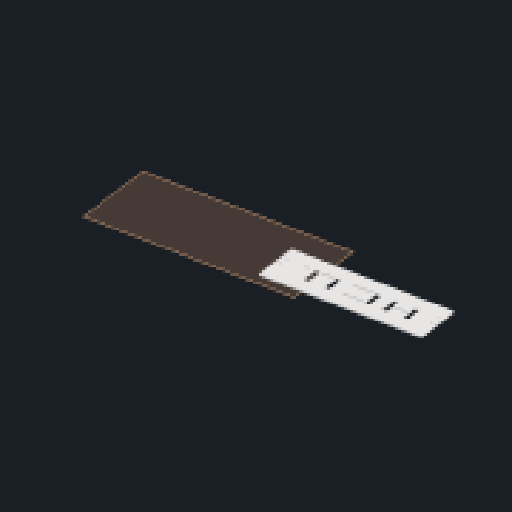
# Autodesk Inventor part: lid
Saved by Autodesk Inventor 2026.1 (Build 301233000, 233)
## iProperties
Created: 2025-08-11
Part Number: lid
Material: Generic
Document SubType Name: Modeling
Designer: jasper
Density: 1 g/cm^3
Appearance: Default
Author: jasper
Autodesk Inventor part; units mm, degrees
ref_plane "YZ Plane" through (0, 0, 0) normal (1, 0, 0) x (0, 1, 0)
ref_plane "XZ Plane" through (0, 0, 0) normal (0, 1, 0) x (-1, 0, 0)
ref_plane "XY Plane" through (0, 0, 0) normal (0, 0, 1) x (1, 0, 0)
ref_plane "Work Plane1" through (-44.2442, 201.0353, -515.4022) normal (0, -0.9118117, 0.4106085) x (-0.1431647, -0.4063788, -0.902419)
sketch "Sketch1" plane through (-44.2442, 201.0353, -515.4022) normal (0, -0.9118117, 0.4106085) x (-0.1431647, -0.4063788, -0.902419)
  circle A0 centre (-31.8295, -172.2882) radius 2.1 projected
  circle A1 centre (-6.35, -6.35) radius 2.1 projected
  circle A2 centre (-31.75, -6.35) radius 2.1 projected
  circle A3 centre (-6.4295, -172.2882) radius 2.1 projected
  circle A4 centre (-31.8295, -172.2882) radius 2.1 projected
  line L0 (50.8, 0) -> (-69.85, 0)
  line L1 (-69.85, 0) -> (-69.85, -178.6382)
  line L2 (-69.85, -178.6382) -> (50.8, -178.6382)
  line L3 (50.8, -178.6382) -> (50.8, 0)
  line L4 (-6.35, -6.35) -> (-31.75, -6.35) construction
  line L5 (-19.05, -6.35) -> (-19.05, -172.2882) construction
  line L6 (-6.4295, -172.2882) -> (-31.8295, -172.2882) construction
  point P0 (-389.7465, -11.674)
  dimension "d41" = 69.85
  dimension "d42" = 50.8
  dimension "d43" = 6.35
  dimension "d44" = 6.35
  constraints: 14 end point, 3 horizontal, 2 parallel, 1 midpoint, 1 perpendicular, 1 point on line, 1 vertical
  measures "d41" distance between parallel lines of L3 L5
  measures "d42" distance between parallel lines of L1 L5
  measures "d43" distance between parallel lines of L4 L0
  measures "d44" distance from line of L2 L6.start
extrude "Extrusion1" add sketch "Sketch1" along normal blind 1.5875
sketch "Sketch2" plane through (-44.2442, 199.5878, -514.7504) normal (0, -0.9118117, 0.4106085) x (-0.9896989, 0.0587846, 0.1305393)
  line L0 (27.0256, 12.7) -> (32.1056, 12.7)
  line L1 (32.1056, 12.7) -> (32.1056, -31.75)
  line L2 (32.1056, -31.75) -> (27.0256, -31.75)
  line L3 (27.0256, -31.75) -> (27.0256, 12.7)
  line L4 (49.8856, 12.7) -> (54.9656, 12.7)
  line L5 (54.9656, 12.7) -> (54.9656, -31.75)
  line L6 (54.9656, -31.75) -> (49.8856, -31.75)
  line L7 (49.8856, -31.75) -> (49.8856, 12.7)
  line L8 (34.6456, -6.985) -> (47.3456, -6.985)
  line L9 (47.3456, -6.985) -> (47.3456, -12.065)
  line L10 (47.3456, -12.065) -> (34.6456, -12.065)
  line L11 (34.6456, -12.065) -> (34.6456, -6.985)
  line L12 (68.9356, 12.7) -> (74.0156, 12.7)
  line L13 (74.0156, 12.7) -> (74.0156, -31.75)
  line L14 (74.0156, -31.75) -> (68.9356, -31.75)
  line L15 (68.9356, -31.75) -> (68.9356, 12.7)
  line L16 (76.5556, 12.7) -> (98.6536, 12.7)
  line L17 (98.6536, 12.7) -> (98.6536, 7.62)
  line L18 (98.6536, 7.62) -> (76.5556, 7.62)
  line L19 (76.5556, 7.62) -> (76.5556, 12.7)
  line L20 (76.5556, -31.75) -> (98.6536, -31.75)
  line L21 (98.6536, -31.75) -> (98.6536, -26.67)
  line L22 (98.6536, -26.67) -> (76.5556, -26.67)
  line L23 (76.5556, -26.67) -> (76.5556, -31.75)
  line L24 (112.6236, 12.7) -> (117.7036, 12.7)
  line L25 (117.7036, 12.7) -> (117.7036, -31.75)
  line L26 (117.7036, -31.75) -> (112.6236, -31.75)
  line L27 (112.6236, -31.75) -> (112.6236, 12.7)
  line L28 (135.4836, 12.7) -> (140.5636, 12.7)
  line L29 (140.5636, 12.7) -> (140.5636, -31.75)
  line L30 (140.5636, -31.75) -> (135.4836, -31.75)
  line L31 (135.4836, -31.75) -> (135.4836, 12.7)
  line L32 (120.2436, -26.67) -> (132.9436, -26.67)
  line L33 (132.9436, -26.67) -> (132.9436, -31.75)
  line L34 (132.9436, -31.75) -> (120.2436, -31.75)
  line L35 (120.2436, -31.75) -> (120.2436, -26.67)
  line L36 (146.5326, -26.67) -> (151.6126, -26.67)
  line L37 (151.6126, -26.67) -> (151.6126, -31.75)
  line L38 (151.6126, -31.75) -> (146.5326, -31.75)
  line L39 (146.5326, -31.75) -> (146.5326, -26.67)
  line L40 (27.0256, -43.4347) -> (151.6126, -43.4347) construction
  line L41 (0, -69.85) -> (178.6382, -69.85) projected
  line L42 (89.3191, -69.85) -> (89.3191, 50.8) construction
  line L43 (178.6382, 50.8) -> (0, 50.8) projected
  line L44 (0, 50.8) -> (0, -69.85) projected
  line L45 (0, -9.525) -> (178.6382, -9.525) construction
  line L46 (178.6382, -69.85) -> (178.6382, 50.8) projected
  point P0 (11.674, -389.7465)
  point P1 (47.3456, -9.525)
  point P2 (34.6456, -9.525)
  point P3 (32.1056, -9.525)
  point P4 (54.9656, -9.525)
  point P5 (132.9436, -29.21)
  point P6 (120.2436, -29.21)
  point P7 (140.5636, -9.525)
  point P8 (89.3191, -43.4347)
  point P9 (12.8847, -9.525)
  dimension "d11" = 5.08
  dimension "d12" = 44.45
  dimension "d13" = 5.08
  dimension "d14" = 44.45
  dimension "d15" = 2.54
  dimension "d16" = 2.54
  dimension "d17" = 12.7
  dimension "d18" = 5.08
  dimension "d19" = 44.45
  dimension "d20" = 13.97
  dimension "d21" = 2.54
  dimension "d22" = 22.098
  dimension "d23" = 5.08
  dimension "d24" = 5.08
  dimension "d25" = 5.08
  dimension "d26" = 44.45
  dimension "d27" = 5.08
  dimension "d28" = 44.45
  dimension "d29" = 2.54
  dimension "d30" = 2.54
  dimension "d31" = 12.7
  dimension "d32" = 5.08
  dimension "d33" = 5.08
  dimension "d34" = 13.97
  dimension "d35" = 5.08
  dimension "d36" = 5.08
  dimension "d37" = 5.969
  constraints: 86 end point, 21 parallel, 12 midpoint, 11 horizontal, 10 perpendicular, 8 collinear, 5 point on line, 2 horizontal alignment
  measures "d11" distance of L0.start L0.end
  measures "d12" distance of L2.end L0.start
  measures "d13" distance of L4.start L4.end
  measures "d14" distance of L6.end L4.start
  measures "d15" distance from line of L7 point (47.346, -9.525)
  measures "d16" distance from line of L1 point (34.646, -9.525)
  measures "d17" distance of L9.end L10.end
  measures "d18" distance of L15.end L13.start
  measures "d19" distance of L14.end L15.end
  measures "d20" distance from line of point (54.966, -9.525) L15
  measures "d21" distance between parallel lines of L13 L19
  measures "d22" distance of L16.start L16.end
  measures "d23" distance of L16.end L17.end
  measures "d24" distance of L20.end L21.end
  measures "d25" distance of L27.end L25.start
  measures "d26" distance of L26.end L27.end
  measures "d27" distance of L28.start L28.end
  measures "d28" distance of L30.end L28.start
  measures "d29" distance from line of L31 point (132.944, -29.21)
  measures "d30" distance from line of L25 point (120.244, -29.21)
  measures "d31" distance of L34.start L34.end
  measures "d32" distance between parallel lines of L34 L32
  measures "d33" distance of L10.end L8.start
  measures "d34" distance between parallel lines of L17 L27
  measures "d35" distance of L36.end L37.end
  measures "d36" distance of L36.start L36.end
  measures "d37" distance between parallel lines of L29 L39
extrude "Extrusion2" cut sketch "Sketch2" against normal blind 1.5875 contours L0 L1 L2 L3 | L4 L5 L6 L7 | L8 L9 L10 L11 | L12 L13 L14 L15 | L16 L17 L18 L19 | L23 L22 L21 L20 | L24 L25 L26 L27 | L28 L29 L30 L31 | L32 L33 L34 L35 | L36 L37 L38 L39
fillet "Fillet2" radius 3.175 4 edges at (-51.517, 179.6675, -560.9192) (-228.315, 190.1686, -537.5999) (-34.2442, 228.6971, -452.0423) (-211.0422, 239.1982, -428.723)
body "Solid1"
